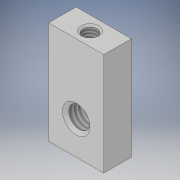
# Autodesk Inventor part: Rear Leg
Saved by Autodesk Inventor 2019.4 (Build 234330000, 330)
## iProperties
Created: 2020-05-07
Part Number: Rear Leg
Material: Generic
Document SubType Name: Modeling
Designer: Workshop Tech
Density: 1 g/cm^3
Appearance: Default
Author: Workshop Tech
Autodesk Inventor part; units mm, degrees
ref_plane "YZ Plane" through (0, 0, 0) normal (1, 0, 0) x (0, 1, 0)
ref_plane "XZ Plane" through (0, 0, 0) normal (0, 1, 0) x (-1, 0, 0)
ref_plane "XY Plane" through (0, 0, 0) normal (0, 0, 1) x (1, 0, 0)
sketch "Sketch1" plane through (0, 0, 0) normal (0, 0, 1) x (1, 0, 0)
  line L0 (0, 0) -> (12.7, 0)
  line L1 (12.7, 0) -> (12.7, 23.622)
  line L2 (12.7, 23.622) -> (0, 23.622)
  line L3 (0, 23.622) -> (0, 0)
  dimension "d0" = 12.7
  dimension "d1" = 23.622
  constraints: 8 end point, 2 parallel, 1 horizontal, 1 perpendicular
  measures "d0" distance between parallel lines of L1 L3
  measures "d1" distance between parallel lines of L0 L2
extrude "Extrusion1" add sketch "Sketch1" along normal blind 6.35
sketch "Sketch2" plane through (0, 0, 6.35) normal (0, 0, 1) x (1, 0, 0)
  line L0 (12.7, 0) -> (12.7, 23.622) projected
  line L1 (0, 0) -> (12.7, 0) projected
  point P0 (6.35, 7.62)
  dimension "d4" = 6.35
  dimension "d5" = 7.62
  measures "d4" distance from line of L0 point (6.35, 7.62)
  measures "d5" distance from line of L1 point (6.35, 7.62)
hole "6 MM Hole" at (6.35, 7.62, 6.35) direction (0, 0, -1) diameter 4.9276 end through all countersink diameter 6.35 countersink angle 90
sketch "Sketch3" plane through (0, 23.622, 0) normal (0, 1, 0) x (1, 0, 0)
  line L0 (12.7, 0) -> (0, 0) projected
  line L1 (0, 0) -> (0, -6.35) projected
  point P0 (6.35, -3.175)
  dimension "d13" = 3.175
  dimension "d14" = 6.35
  measures "d13" distance from line of L0 point (6.35, -3.175)
  measures "d14" distance from line of L1 point (6.35, -3.175)
hole "Hole2" at (6.35, 23.622, 3.175) direction (0, -1, 0) diameter 3.2512 depth 12.065 tip angle 118 countersink diameter 4.064 countersink angle 90
chamfer "Chamfer1" distance 0.508 angle 45 1 edges at (6.35, 10.0838, 0)
body "Solid1"
